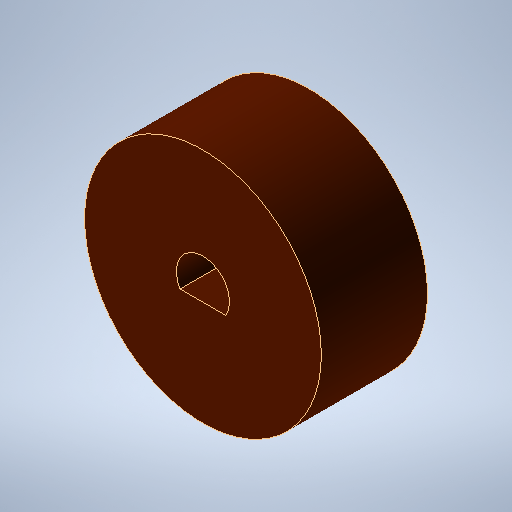
# Autodesk Inventor part: Tlacitko
Saved by Autodesk Inventor 2025.2 (Build 292293000, 293)
## iProperties
Created: 2025-03-26
Part Number: Tlacitko
Material: Všeobecné
Document SubType Name: Modeling
Designer: jakub
Density: 1 g/cm^3
Appearance: Oranžová
Author: jakub
## iProperties of the stored document Tlacitko_3D tisk.ipt
Created: 2025-03-26
Part Number: Tlacitko_3D tisk
Material: Všeobecné
Document SubType Name: Modeling
Designer: jakub
Density: 1 g/cm^3
Appearance: Výchozí
Author: jakub
Autodesk Inventor part; units mm, degrees
ref_plane "YZ Plane" through (0, 0, 0) normal (1, 0, 0) x (0, 1, 0)
ref_plane "XZ Plane" through (0, 0, 0) normal (0, 1, 0) x (-1, 0, 0)
ref_plane "XY Plane" through (0, 0, 0) normal (0, 0, 1) x (1, 0, 0)
sketch "Náčrt1" plane through (0, 0, 0) normal (0, 0, 1) x (1, 0, 0)
  line L0 (0, 20.3) -> (0, -20.3) projected
  line L1 (-20.3, 0) -> (20.3, 0) projected
  circle A0 centre (0, 0) radius 14.5
  dimension "d0" = 29
  constraints: 1 centre point, 1 coincident
  measures "d0" diameter of A0
extrude "Vysunutí1" add sketch "Náčrt1" along normal blind 13
sketch "Náčrt2" plane through (0, 0, 13) normal (0, 0, 1) x (1, 0, 0)
  line L0 (0, 20.3) -> (0, -20.3) projected
  line L1 (-20.3, 0) -> (20.3, 0) projected
  arc A0 (2.8, -1.65) -> (-2.8, -1.65) centre (0, 0) ccw
  line L2 (-2.8, -1.65) -> (2.8, -1.65)
  dimension "d3" = 6.5
  dimension "d4" = 4.9
  constraints: 2 end point, 2 point on circle, 1 centre point, 1 coincident, 1 horizontal
  measures "d3" diameter of A0
extrude "Vysunutí2" cut sketch "Náčrt2" against normal blind 11
